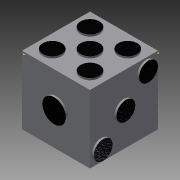
# Autodesk Inventor part: dicemodel1
Saved by Autodesk Inventor 2015 (Build 190159000, 159)
## iProperties
Created: 2018-01-15
Part Number: dicemodel1
Material: Generic
Document SubType Name: Modeling
Designer: Alex
Density: 1 g/cm^3
Appearance: Default
Author: Alex
Autodesk Inventor part; units mm, degrees
ref_plane "YZ Plane" through (0, 0, 0) normal (1, 0, 0) x (0, 1, 0)
ref_plane "XZ Plane" through (0, 0, 0) normal (0, 1, 0) x (-1, 0, 0)
sketch "Sketch1" plane through (0, 0, 0) normal (0, 0, 1) x (1, 0, 0)
  line L0 (-13.4099, 13.8043) -> (443.7901, 13.8043)
  line L1 (443.7901, 13.8043) -> (443.7901, -443.3957)
  line L2 (443.7901, -443.3957) -> (-13.4099, -443.3957)
  line L3 (-13.4099, -443.3957) -> (-13.4099, 13.8043)
  point P0 (0, 0)
  dimension "d0" = 457.2
  dimension "d1" = 457.2
  constraints: 8 end point, 2 parallel, 1 horizontal, 1 perpendicular
  measures "d0" distance of L0.start L0.end
  measures "d1" distance of L2.end L0.start
extrude "Extrusion1" add sketch "Sketch1" along normal blind 457.2
ref_plane "Work Plane1" through (443.7901, 0, 457.2) normal (-0.7071, 0, 0.7071) x (0, -1, 0)
sketch "Sketch2" plane through (0, 0, 457.2) normal (0, 0, 1) x (1, 0, 0)
  point P0 (0, 0)
sketch "Sketch3" plane through (0, 0, 457.2) normal (0, 0, 1) x (1, 0, 0)
  circle A0 centre (215.1901, -214.7957) radius 78.8174
  line L0 (443.7901, -443.3957) -> (443.7901, 13.8043) projected
  line L1 (443.7901, 13.8043) -> (-13.4099, 13.8043) projected
  point P0 (0, 0)
  dimension "d4" = 228.6
  dimension "d5" = 228.6
  constraints: 1 centre point
  measures "d4" distance from line of L0 A0.centre
  measures "d5" distance from line of L1 A0.centre
extrude "Extrusion2" add sketch "Sketch3" along normal blind 12.7
sketch "Sketch4" plane through (443.7901, -443.3957, 0) normal (1, 0, 0) x (0, 0, -1)
  point P0 (0, 443.3957)
sketch "Sketch5" plane through (443.7901, -443.3957, 0) normal (1, 0, 0) x (0, 0, -1)
  line L0 (0, 457.2) -> (-457.2, 0)
  circle A0 centre (-76.1993, 381.0007) radius 63.5
  circle A1 centre (-228.6, 228.6) radius 63.5
  circle A2 centre (-381.0007, 76.1993) radius 63.5
  point P0 (0, 443.3957)
  dimension "d21" = 127
  dimension "d22" = 127
  dimension "d23" = 127
  dimension "d25" = 646.5784
  dimension "d26" = 107.762
  dimension "d28" = 107.762
  constraints: 3 centre point, 2 end point, 2 point on line, 1 midpoint
  measures "d21" diameter of A2
  measures "d22" diameter of A1
  measures "d23" diameter of A0
  measures "d25" distance of L0.start L0.end
  measures "d26" distance of L0.start A0.centre
  measures "d28" distance of L0.end A2.centre
extrude "Extrusion3" add sketch "Sketch5" along normal blind 12.7
sketch "Sketch6" plane through (-13.4099, -443.3957, 0) normal (-1, 0, 0) x (0, 0, 1)
  line L0 (0, 457.2) -> (457.2, 0)
  line L1 (114.3, 342.9) -> (342.9, 342.9)
  line L2 (342.9, 342.9) -> (342.9, 114.3)
  line L3 (342.9, 114.3) -> (114.3, 114.3)
  line L4 (114.3, 114.3) -> (114.3, 342.9)
  line L5 (0, 0) -> (0, 457.2) projected
  line L6 (457.2, 457.2) -> (457.2, 0) projected
  circle A0 centre (114.3, 342.9) radius 63.5
  circle A1 centre (342.9, 342.9) radius 63.5
  circle A2 centre (114.3, 114.3) radius 63.5
  circle A3 centre (342.9, 114.3) radius 63.5
  point P0 (228.6, 228.6)
  dimension "d37" = 228.6
  dimension "d38" = 114.3
  dimension "d40" = 127
  dimension "d41" = 127
  dimension "d42" = 127
  dimension "d43" = 127
  constraints: 10 end point, 4 centre point, 4 coincident, 2 parallel, 2 point on line, 1 horizontal, 1 midpoint, 1 perpendicular
  measures "d37" distance of L1.start L1.end
  measures "d38" distance between parallel lines of L5 L4
  measures "d40" diameter of A0
  measures "d41" diameter of A1
  measures "d42" diameter of A3
  measures "d43" diameter of A2
extrude "Extrusion4" add sketch "Sketch6" along normal blind 12.7 contours A0 L1 L0 | L0 L4 A0 | L1 A0 L0 | L0 A0 L4 | A1 L2 L1 | L1 L2 A1 | A2 L3 L4 | L4 L3 A2 | A3 L2 L0 | L0 L3 A3 | L2 A3 L0 | L0 A3 L3
sketch "Sketch7" plane through (0, 0, 0) normal (0, 0, -1) x (-1, 0, 0)
  line L0 (-443.7901, 13.8043) -> (-316.7901, 13.8043)
  line L1 (-443.7901, 13.8043) -> (13.4099, 13.8043) projected
  line L2 (13.4099, 13.8043) -> (-113.5901, 13.8043)
  line L3 (-443.7901, -443.3957) -> (13.4099, -443.3957) projected
  line L4 (-316.7901, 13.8043) -> (-316.7901, -443.3957)
  line L5 (-113.5901, 13.8043) -> (-113.5901, -443.3957)
  line L6 (-316.7901, 13.8043) -> (-316.7901, -62.3957)
  line L7 (-316.7901, -443.3957) -> (-316.7901, -367.1957)
  circle A0 centre (-316.7901, -62.3957) radius 63.5
  circle A1 centre (-316.7901, -367.1957) radius 63.5
  circle A2 centre (-316.7901, -214.7957) radius 63.5
  circle A3 centre (-113.5901, -62.3957) radius 63.5
  circle A4 centre (-113.5901, -214.7957) radius 63.5
  circle A5 centre (-113.5901, -367.1957) radius 63.5
  point P0 (0, 0)
  dimension "d46" = 127
  dimension "d47" = 127
  dimension "d53" = 76.2
  dimension "d54" = 76.2
  dimension "d55" = 127
  dimension "d56" = 127
  dimension "d57" = 127
  dimension "d58" = 127
  dimension "d59" = 127
  dimension "d60" = 127
  constraints: 12 end point, 8 point on line, 6 centre point, 2 coincident, 2 midpoint, 2 perpendicular
  measures "d46" distance of L0.start L0.end
  measures "d47" distance of L1.end L2.end
  measures "d53" distance of L0.end L6.end
  measures "d54" distance of L4.end L7.end
  measures "d55" diameter of A0
  measures "d56" diameter of A2
  measures "d57" diameter of A1
  measures "d58" diameter of A5
  measures "d59" diameter of A4
  measures "d60" diameter of A3
extrude "Extrusion5" add sketch "Sketch7" along normal blind 12.7 contours A0 L4 | L4 A0 | A3 L5 | L5 A3 | A2 L4 | L4 A2 | A4 L5 | L5 A4 | A1 L4 | L4 A1 | A5 L5 | L5 A5
sketch "Sketch8" plane through (-13.4099, 13.8043, 0) normal (0, 1, 0) x (1, 0, 0)
  line L0 (355.6, -101.6) -> (101.6, -101.6)
  line L1 (101.6, -101.6) -> (101.6, -355.6)
  line L2 (101.6, -355.6) -> (355.6, -355.6)
  line L3 (355.6, -355.6) -> (355.6, -101.6)
  line L4 (355.6, -101.6) -> (101.6, -355.6)
  circle A0 centre (355.6, -101.6) radius 63.5
  line L5 (0, 0) -> (457.2, 0) projected
  line L6 (457.2, -457.2) -> (0, -457.2) projected
  line L7 (457.2, 0) -> (457.2, -457.2) projected
  circle A1 centre (228.6, -228.6) radius 63.5
  circle A2 centre (101.6, -101.6) radius 63.5
  circle A3 centre (101.6, -355.6) radius 63.5
  circle A4 centre (355.6, -355.6) radius 63.5
  point P0 (13.4099, 0)
  dimension "d63" = 254
  dimension "d64" = 101.6
  dimension "d65" = 101.6
  dimension "d66" = 101.6
  dimension "d67" = 127
  dimension "d68" = 127
  dimension "d69" = 127
  dimension "d70" = 127
  dimension "d71" = 127
  constraints: 10 end point, 5 centre point, 3 coincident, 2 parallel, 1 horizontal, 1 midpoint, 1 perpendicular
  measures "d63" distance of L2.end L1.end
  measures "d64" distance between parallel lines of L5 L0
  measures "d65" distance between parallel lines of L6 L2
  measures "d66" distance between parallel lines of L7 L3
  measures "d67" diameter of A0
  measures "d68" diameter of A1
  measures "d69" diameter of A2
  measures "d70" diameter of A3
  measures "d71" diameter of A4
extrude "Extrusion6" add sketch "Sketch8" along normal blind 12.7 contours A2 L1 L0 | L0 L1 A2 | A0 L3 L0 | L0 L4 A0 | L3 A0 L4 | A3 L4 L1 | L1 L2 A3 | A1 L4 | L4 A1 | L4 A3 L2 | A4 L2 L3 | L3 L2 A4
sketch "Sketch9" plane through (-13.4099, -443.3957, 0) normal (0, -1, 0) x (1, 0, 0)
  line L0 (0, 0) -> (457.2, 457.2)
  line L1 (457.2, 457.2) -> (304.8, 304.8)
  line L2 (0, 0) -> (152.4, 152.4)
  circle A0 centre (152.4, 152.4) radius 63.5
  circle A1 centre (304.8, 304.8) radius 63.5
  point P0 (13.4099, 0)
  dimension "d77" = 646.5784
  dimension "d78" = 127
  dimension "d79" = 127
  constraints: 6 end point, 2 centre point, 2 coincident, 2 point on line
  measures "d77" distance of L0.start L0.end
  measures "d78" diameter of A0
  measures "d79" diameter of A1
extrude "Extrusion7" add sketch "Sketch9" along normal blind 12.7
body "Solid1"
